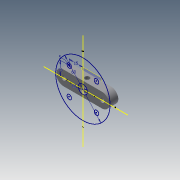
# Autodesk Inventor part: pulleyFlange
Saved by Autodesk Inventor 2015 (Build 190159000, 159)
## iProperties
Created: 2014-09-01
Part Number: pulleyFlange
Material: Generic
Document SubType Name: Modeling
Designer: shohei
Density: 1 g/cm^3
Appearance: Default
Author: shohei
Autodesk Inventor part; units mm, degrees
ref_plane "YZ Plane" through (0, 0, 0) normal (1, 0, 0) x (0, 1, 0)
ref_plane "XZ Plane" through (0, 0, 0) normal (0, 1, 0) x (-1, 0, 0)
ref_plane "XY Plane" through (0, 0, 0) normal (0, 0, 1) x (1, 0, 0)
sketch "Block1" plane through (0, 0, 0) normal (0, 0, 1) x (1, 0, 0)
  circle A0 centre (0, 0) radius 40.22
  circle A1 centre (30, -0.0076) radius 2.22
  circle A2 centre (0.0076, 30) radius 2.22
  circle A3 centre (0, 0) radius 5.22
  circle A4 centre (-30, 0.0076) radius 2.22
  circle A5 centre (-0.0076, -30) radius 2.22
  point P0 (0, 0)
sketch "Block2" plane through (0, 0, 0) normal (0, 0, 1) x (1, 0, 0)
  circle A0 centre (0, 0) radius 20.22
  circle A1 centre (10, -0.0076) radius 2.22
  circle A2 centre (0.0076, 10) radius 2.22
  circle A3 centre (0, 0) radius 5.22
  circle A4 centre (-0.0076, -10) radius 2.22
  circle A5 centre (-10, 0.0076) radius 2.22
  point P0 (0, 0)
sketch "Sketch1" plane through (0, 0, 0) normal (0, 1, 0) x (-1, 0, 0)
  circle A0 centre (0, 0) radius 30
  circle A1 centre (0, 0) radius 5
  arc A2 (-36.0813, 0.572) -> (-36.0815, -0.5576) centre (0, 0) ccw
  arc A3 (-0.0152, -40) -> (-0.0008, -40) centre (0, 0) ccw
  arc A4 (-0.5728, -36.0815) -> (0.5584, -36.0818) centre (0, 0) ccw
  circle A5 centre (15, 15) radius 2.5
  line L0 (43.2172, 0) -> (-49.3032, 0) projected
  line L1 (0, -55.2163) -> (0, 51.2978) projected
  circle A6 centre (15, -15) radius 2.5
  circle A7 centre (-15, 15) radius 2.5
  circle A8 centre (-15, -15) radius 2.5
  point P0 (17, -0.0008)
  point P1 (13.0813, -0.572)
  point P2 (-36.0815, 0.5728)
  point P3 (-0.5576, 36.0815)
  point P4 (0.572, 36.0813)
  point P5 (-13.0813, -0.572)
  dimension "d0" = 60
  dimension "d7" = 10
  dimension "d31" = 5
  dimension "d32" = 15
  dimension "d33" = 15
  constraints: 9 centre point, 6 point on circle, 4 symmetric about line, 3 coincident, 3 other
  measures "d0" diameter of A0
  measures "d7" diameter of A1
  measures "d31" diameter of A5
  measures "d32" distance from line of L0 A5.centre
  measures "d33" distance from line of L1 A5.centre
ref_plane "Work Plane1" through (0, 10, 0) normal (0, 1, 0) x (1, 0, 0)
sketch "Sketch6" plane through (0, 0, 0) normal (0, 1, 0) x (-1, 0, 0)
  line L0 (21.2132, 0) -> (-21.2132, 0) construction
  line L1 (21.2132, 8) -> (-21.2132, 8)
  line L2 (-21.2132, -8) -> (21.2132, -8)
  arc A0 (21.2132, -8) -> (21.2132, 8) centre (21.2132, 0) ccw
  arc A1 (-21.2132, 8) -> (-21.2132, -8) centre (-21.2132, 0) ccw
  circle A2 centre (-21.2132, 0) radius 2.5
  circle A3 centre (21.2132, 0) radius 2.5
  circle A4 centre (0, 0) radius 5
  dimension "d36" = 8
  dimension "d37" = 5
  dimension "d38" = 5
  dimension "d39" = 42.4264
  dimension "d40" = 10
  constraints: 8 end point, 5 centre point, 4 point on circle, 4 tangent, 3 coincident, 1 horizontal, 1 midpoint, 1 parallel
  measures "d36" radius of A1
  measures "d37" diameter of A2
  measures "d38" diameter of A3
  measures "d39" distance of L2.start L2.end
  measures "d40" diameter of A4
extrude "Extrusion4" add sketch "Sketch6" along normal blind 10
sketch "Sketch7" plane through (21.2132, 0, -8) normal (0, 0, -1) x (-1, 0, 0)
  circle A0 centre (21.2132, 5) radius 2.5
  line L0 (0, 10) -> (42.4264, 10) projected
  line L1 (0, 0) -> (0, 10) projected
  point P0 (21.2132, 0)
  dimension "d43" = 5
  dimension "d44" = 5
  dimension "d45" = 21.2132
  constraints: 1 centre point
  measures "d43" diameter of A0
  measures "d44" distance from line of L0 A0.centre
  measures "d45" distance from line of L1 A0.centre
extrude "Extrusion5" cut sketch "Sketch7" against normal through all
body "Solid4"
